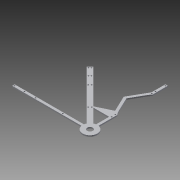
# Autodesk Inventor part: Bearing Mount Top
Saved by Autodesk Inventor 2013 (Build 170138000, 138)
## iProperties
Created: 2013-01-21
Part Number: Bearing Mount Top
Material: Aluminum 6061
Document SubType Name: Modeling
Designer: actoennies
Mass: 423.201 g
Surface Area: 681.787 cm^2
Volume: 156.163 cm^3
Density: 2.71 g/cm^3
Author: actoennies
Autodesk Inventor part; units mm, degrees
ref_plane "YZ Plane" through (0, 0, 0) normal (1, 0, 0) x (0, 1, 0)
ref_plane "XZ Plane" through (0, 0, 0) normal (0, 1, 0) x (-1, 0, 0)
ref_plane "XY Plane" through (0, 0, 0) normal (0, 0, 1) x (1, 0, 0)
sketch "Sketch1" plane through (0, 0, 0) normal (0, 1, 0) x (-1, 0, 0)
  circle A0 centre (0, -139.7) radius 3.3782
  line L0 (6.35, -37.5671) -> (6.35, -393.6488)
  line L1 (-6.35, -37.5671) -> (-6.35, -393.7)
  circle A1 centre (193.0245, -202.0047) radius 3.3782
  circle A2 centre (202.0047, -193.0245) radius 3.3782
  line L2 (269.2628, -287.2233) -> (16.4197, -34.3803)
  line L3 (287.2233, -269.2628) -> (34.3803, -16.4197)
  circle A3 centre (94.1906, -103.1708) radius 3.3782
  circle A4 centre (103.1708, -94.1906) radius 3.3782
  circle A5 centre (139.7, 0) radius 3.3782
  line L4 (133.35, 0) -> (133.35, 6.35)
  line L5 (273.05, 6.35) -> (273.05, 0)
  line L6 (37.5671, -6.35) -> (393.6488, -6.35)
  line L7 (37.5671, 6.35) -> (393.7, 6.35)
  line L8 (146.05, 0) -> (146.05, 6.35)
  circle A6 centre (277.5195, -270.2276) radius 3.3782
  circle A7 centre (270.2276, -277.5195) radius 3.3782
  arc A8 (269.2628, -287.2233) -> (287.2233, -269.2628) centre (0, 0) ccw
  circle A9 centre (0, -387.35) radius 3.3782
  arc A10 (0, -393.7) -> (6.35, -393.6488) centre (0, 0) ccw
  line L9 (-6.35, -393.7) -> (0, -393.7)
  circle A11 centre (0, -279.4) radius 3.3782
  arc A12 (6.35, -37.5671) -> (16.4197, -34.3803) centre (0, 0) ccw
  arc A13 (34.3803, -16.4197) -> (37.5671, -6.35) centre (0, 0) ccw
  circle A14 centre (0, 0) radius 14.2875
  line L10 (38.1, 0) -> (38.1, 12.8556) construction
  arc A15 (-6.214, 37.5898) -> (-37.5898, 6.214) centre (0, 0) ccw
  arc A16 (37.5671, 6.35) -> (-6.35, -37.5671) centre (0, 0) ccw
  circle A17 centre (387.35, 0) radius 3.3782
  line L11 (393.7, 0) -> (393.7, 6.35)
  circle A18 centre (279.4, 0) radius 3.3782
  line L12 (285.75, 6.35) -> (285.75, 0)
  arc A19 (393.6488, -6.35) -> (393.7, 0) centre (0, 0) ccw
  line L13 (0, -285.75) -> (-6.35, -285.75)
  line L14 (-6.35, -273.05) -> (0, -273.05)
  circle A20 centre (0, -336.55) radius 3.3782
  circle A21 centre (241.5985, -234.3065) radius 3.3782
  circle A22 centre (234.3065, -241.5985) radius 3.3782
  circle A23 centre (336.55, 0) radius 3.3782
  dimension "d2" = 12.7
  dimension "d3" = 12.7
  dimension "d4" = 38.1
  dimension "d6" = 38.1
  dimension "d7" = 6.35
  dimension "d8" = 6.35
  dimension "d9" = 6.35
  dimension "d10" = 12.7
  dimension "d11" = 12.7
  dimension "d12" = 95.25
  dimension "d13" = 6.7564
  dimension "d14" = 6.7564
  dimension "d15" = 6.7564
  dimension "d16" = 6.35
  dimension "d17" = 6.7564
  dimension "d18" = 6.35
  dimension "d19" = 6.35
  dimension "d20" = 6.7564
  dimension "d21" = 6.7564
  dimension "d22" = 6.7564
  dimension "d23" = 6.35
  dimension "d24" = 6.7564
  dimension "d25" = 28.575
  dimension "d28" = 38.1
  dimension "d30" = 6.35
  dimension "d31" = 139.7
  dimension "d34" = 6.35
  dimension "d37" = 277.5195
  dimension "d38" = 270.2276
  dimension "d39" = 7.2919
  dimension "d40" = 7.2919
  dimension "d41" = 393.7
  dimension "d42" = 393.7
  dimension "d43" = 6.35
  dimension "d44" = 12.7
  dimension "d45" = 6.7564
  dimension "d46" = 6.35
  dimension "d47" = 6.7564
  dimension "d48" = 6.7564
  dimension "d49" = 393.7
  dimension "d50" = 6.35
  dimension "d51" = 6.7564
  dimension "d52" = 6.35
  dimension "d54" = 6.7564
  dimension "d55" = 6.7564
  dimension "d56" = 6.7564
  dimension "d57" = 50.8
  dimension "d58" = 50.8
  dimension "d59" = 50.8
  dimension "d60" = 7.5438
  dimension "d61" = 7.5438
  dimension "d62" = 7.5438
  dimension "d63" = 7.5438
  dimension "d64" = 50.8
  constraints: 30 end point, 24 centre point, 15 point on circle, 6 point on line, 5 perpendicular, 4 parallel
  measures "d2" distance from line of L2 A10.centre
  measures "d3" distance from line of A10.centre L3
  measures "d4" radius of A15
  measures "d6" radius of A12
  measures "d7" distance from line of L1 A10.centre
  measures "d8" distance from line of A10.centre L0
  measures "d9" distance from line of L7 A10.centre
  measures "d10" distance between parallel lines of L8 L4
  measures "d11" distance between parallel lines of L5 L12
  measures "d12" distance from line of L4 L10.start
  measures "d13" diameter of A4
  measures "d14" diameter of A3
  measures "d15" diameter of A18
  measures "d16" distance from line of L7 A18.centre
  measures "d17" diameter of A5
  measures "d18" distance from line of L7 A5.centre
  measures "d19" distance from line of L8 A5.centre
  measures "d20" diameter of A2
  measures "d21" diameter of A1
  measures "d22" diameter of A11
  measures "d23" distance from line of L1 A11.centre
  measures "d24" diameter of A0
  measures "d25" diameter of A14
  measures "d28" radius of A13
  measures "d30" distance from line of point (0, 0) L1
  measures "d31" distance of point (0, 0) A0.centre
  measures "d34" distance from line of L0 A9.centre
  measures "d37" vertical distance of A10.centre A7.centre
  measures "d38" horizontal distance of point (0, 0) A7.centre
  measures "d39" horizontal distance of A7.centre A6.centre
  measures "d40" horizontal distance of A7.centre A6.centre
  measures "d41" radius of A8
  measures "d42" radius of A19
  measures "d43" distance of L11.start L7.end
  measures "d44" distance between parallel lines of L6 L7
  measures "d45" diameter of A17
  measures "d46" distance from line of L6 A17.centre
  measures "d47" diameter of A6
  measures "d48" diameter of A7
  measures "d49" radius of A10
  measures "d50" distance of L1.end L9.end
  measures "d51" diameter of A20
  measures "d52" distance of L9.end A9.centre
  measures "d54" diameter of A21
  measures "d55" diameter of A22
  measures "d56" diameter of A23
  measures "d57" distance of A17.centre A23.centre
  measures "d58" distance of A6.centre A21.centre
  measures "d59" distance of A7.centre A22.centre
  measures "d60" distance from line of L3 A21.centre
  measures "d61" distance from line of L2 A22.centre
  measures "d62" distance from line of L2 A7.centre
  measures "d63" distance from line of L3 A6.centre
  measures "d64" distance of A20.centre A9.centre
extrude "Extrusion1" add sketch "Sketch1" along normal blind 6.35
sketch "Sketch3" plane through (0, 6.35, 0) normal (0, 1, 0) x (1, 0, 0)
  circle A0 centre (0, 139.7) radius 3.3782 projected
  circle A1 centre (0, 279.4) radius 3.3782 projected
  arc A2 (114.1705, 370.2558) -> (114.1705, 78.432) centre (120.5205, 224.3439) ccw projected
  circle A3 centre (120.5205, 224.3439) radius 146.05
  circle A4 centre (0, 139.7) radius 3.3782
  constraints: 2 coincident, 1 centre point, 1 concentric, 3 other
extrude "Extrusion2" cut sketch "Sketch3" against normal blind 25.4 contours A0 A2 | A0 A2 A3 picked at (1.5488, 140.8748)
sketch "Sketch4" plane through (0, 6.35, 0) normal (0, 1, 0) x (1, 0, 0)
  arc A0 (-0.7723, 142.9887) -> (2.8315, 137.8575) centre (0, 139.7) ccw projected
  line L0 (-0.7723, 142.9887) -> (2.8315, 137.8575)
  constraints: 2 end point
extrude "Extrusion3" add sketch "Sketch4" against normal blind 6.35
sketch "Sketch5" plane through (0, 6.35, 0) normal (0, 1, 0) x (1, 0, 0)
  arc A0 (-6.35, 37.5671) -> (-16.4197, 34.3803) centre (0, 0) ccw projected
  circle A1 centre (95.9038, 387.35) radius 3.3782 projected
  line L0 (-33.7845, 268.7939) -> (-50.9295, 268.7939) projected
  line L1 (-50.9295, 268.7939) -> (-50.9295, 239.5157) projected
  line L2 (-50.9295, 239.5157) -> (-33.7845, 239.5157) projected
  line L3 (-33.7845, 239.5157) -> (-33.7845, 234.4357) projected
  line L4 (-33.7845, 234.4357) -> (-50.9295, 224.3439) projected
  arc A2 (-50.9295, 224.3439) -> (114.1705, 53.0115) centre (120.5205, 224.3439) ccw projected
  line L5 (114.1705, 53.0115) -> (114.1705, 63.0539) projected
  line L6 (114.1705, 63.0539) -> (128.1405, 63.0539) projected
  line L7 (128.1405, 63.0539) -> (128.1405, 73.2139) projected
  line L8 (128.1405, 73.2139) -> (114.1705, 73.2139) projected
  line L9 (114.1705, 73.2139) -> (114.1705, 78.432) projected
  arc A3 (114.1705, 370.2558) -> (114.1705, 78.432) centre (120.5205, 224.3439) ccw projected
  line L10 (114.1705, 370.2558) -> (114.1705, 375.4739) projected
  line L11 (114.1705, 375.4739) -> (128.1405, 375.4739) projected
  line L12 (128.1405, 375.4739) -> (128.1405, 385.6339) projected
  line L13 (128.1405, 385.6339) -> (114.1705, 385.6339) projected
  line L14 (114.1705, 385.6339) -> (114.1705, 395.6763) projected
  arc A4 (114.1705, 395.6763) -> (-33.7845, 299.0772) centre (120.5205, 224.3439) ccw projected
  line L15 (-33.7845, 299.0772) -> (-33.7845, 268.7939) projected
  line L16 (-43.3095, 256.7035) -> (-33.7845, 256.7035) projected
  line L17 (-33.7845, 256.7035) -> (-33.7845, 246.5435) projected
  line L18 (-33.7845, 246.5435) -> (-43.3095, 246.5435) projected
  line L19 (-43.3095, 246.5435) -> (-43.3095, 256.7035) projected
  circle A5 centre (0, 111.125) radius 3.3782
  circle A6 centre (0, 130.175) radius 3.3782
  circle A7 centre (0, 336.55) radius 3.3782 projected
  circle A8 centre (0, 317.5) radius 3.3782
  circle A9 centre (0, 130.175) radius 3.3782 projected
  circle A10 centre (0, 317.5) radius 3.3782 projected
  circle A11 centre (0, 336.55) radius 3.3782 projected
  circle A12 centre (0, 111.125) radius 3.3782 projected
  dimension "d81" = 6.7564
  dimension "d82" = 6.7564
  dimension "d83" = 6.7564
  dimension "d84" = 19.05
  dimension "d85" = 19.05
  dimension "d86" = 111.125
  constraints: 3 centre point
  measures "d81" diameter of A5
  measures "d82" diameter of A6
  measures "d83" diameter of A8
  measures "d84" distance of A7.centre A8.centre
  measures "d85" distance of A6.centre A5.centre
  measures "d86" distance of A5.centre A0.centre
extrude "Extrusion4" cut sketch "Sketch5" against normal blind 2540 contours A5 | A6 | A8
sketch "Sketch6" plane through (0, 6.35, 0) normal (0, 1, 0) x (1, 0, 0)
  circle A0 centre (0, 111.125) radius 3.3782 projected
  line L0 (-6.35, 151.9942) -> (-6.35, 37.5671) projected
  line L1 (-16.4197, 34.3803) -> (-269.2628, 287.2233) projected
  circle A1 centre (-94.1906, 103.1708) radius 3.3782 projected
  line L2 (-23.9902, 155.9303) -> (-93.3223, 111.2828)
  circle A2 centre (0, 317.5) radius 3.3782 projected
  circle A3 centre (0, 387.35) radius 3.3782 projected
  circle A4 centre (0, 336.55) radius 3.3782 projected
  arc A5 (6.35, 315.4246) -> (-6.35, 296.6936) centre (120.5205, 224.3439) ccw projected
  line L3 (6.35, 315.4246) -> (6.35, 393.7) projected
  line L4 (6.35, 393.7) -> (0, 393.7) projected
  arc A6 (0, 393.7) -> (-6.35, 393.6488) centre (0, 0) ccw projected
  line L5 (-6.35, 393.6488) -> (-6.35, 296.6936) projected
  line L6 (-57.15, 230.8802) -> (-6.35, 151.9942)
  line L7 (-71.4175, 229.5789) -> (-23.9902, 155.9303)
  line L8 (-6.35, 104.2162) -> (-80.0333, 97.9938)
  line L9 (-57.15, 230.8802) -> (-6.35, 296.6936)
  line L10 (-71.4175, 229.5789) -> (-6.35, 313.8765)
  point P0 (-86.8145, 104.775)
  point P1 (-6.35, 322.3307)
  dimension "d90" = 6.35
  dimension "d94" = 12.7
  dimension "d95" = 50.8
  dimension "d96" = 6.35
  dimension "d97" = 6.35
  constraints: 12 end point, 6 point on line, 2 parallel, 1 perpendicular
  measures "d90" distance from line of A1.centre L2
  measures "d94" distance between parallel lines of L7 L6
  measures "d95" horizontal distance of L6.start L0.start
  measures "d96" distance from line of A0.centre L8
  measures "d97" distance from line of A1.centre L8
extrude "Extrusion5" add sketch "Sketch6" against normal blind 6.35 contours L0 L8 L1 L2 L7 L10 L5 L9 L6
equation "\"d60\" = d63"
equation "\"d61\" = d62"
body "Solid1"
